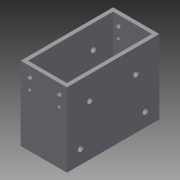
# Autodesk Inventor part: Pitch_Free_Case
Saved by Autodesk Inventor 2013 (Build 170138000, 138)
## iProperties
Created: 2014-05-25
Part Number: Pitch_Free_Case
Material: 一般
Document SubType Name: Modeling
Designer: andou
Density: 1 g/cm^3
Author: andou
Autodesk Inventor part; units mm, degrees
ref_plane "YZ Plane" through (0, 0, 0) normal (1, 0, 0) x (0, 1, 0)
ref_plane "XZ Plane" through (0, 0, 0) normal (0, 1, 0) x (-1, 0, 0)
ref_plane "XY Plane" through (0, 0, 0) normal (0, 0, 1) x (1, 0, 0)
sketch "スケッチ1" plane through (0, 0, 0) normal (0, 0, 1) x (1, 0, 0)
  line L0 (-12.5, 25) -> (12.5, 25)
  line L1 (12.5, 25) -> (12.5, -25)
  line L2 (12.5, -25) -> (-12.5, -25)
  line L3 (-12.5, -25) -> (-12.5, 25)
  line L4 (-10.5, 23) -> (10.5, 23)
  line L5 (10.5, 23) -> (10.5, -23)
  line L6 (10.5, -23) -> (-10.5, -23)
  line L7 (-10.5, -23) -> (-10.5, 23)
  point P0 (0, 0)
  dimension "d0" = 21
  dimension "d2" = 25
  dimension "d3" = 10.5
  dimension "d4" = 46
  dimension "d5" = 50
  dimension "d6" = 23
  dimension "d7" = 25
  dimension "d8" = 12.5
  constraints: 16 end point, 4 parallel, 2 horizontal, 2 perpendicular
  measures "d0" distance of L4.start L4.end
  measures "d2" distance of L0.start L0.end
  measures "d3" distance from line of L7 point (0, 0)
  measures "d4" distance between parallel lines of L6 L4
  measures "d5" distance of L2.end L0.start
  measures "d6" distance from line of point (0, 0) L6
  measures "d7" distance from line of point (0, 0) L2
  measures "d8" distance from line of L1 point (0, 0)
extrude "押し出し1" add sketch "スケッチ1" against normal blind 40
sketch "スケッチ2" plane through (-12.5, 25, 0) normal (0, 1, 0) x (1, 0, 0)
  line L0 (0, 0) -> (25, 0) projected
  line L1 (0, 0) -> (0, 40) projected
  circle A0 centre (4.5, 5) radius 1.5
  circle A1 centre (20.5, 5) radius 1.5
  point P0 (12.5, 0)
  dimension "d13" = 3
  dimension "d14" = 16
  dimension "d16" = 4.5
  dimension "d18" = 5
  dimension "d21" = 5
  constraints: 2 centre point, 1 equal radius
  measures "d13" diameter of A0
  measures "d14" distance of A1.centre A0.centre
  measures "d16" distance from line of L1 A0.centre
  measures "d18" distance from line of L0 A0.centre
  measures "d21" distance from line of A1.centre L0
hole "穴1" at (8, 25, -5) at (-8, 25, -5) direction (0, -1, 0) diameter 3 end through all
sketch "スケッチ3" plane through (-12.5, 25, 0) normal (0, 1, 0) x (1, 0, 0)
  circle A0 centre (20.5, 5) radius 1.5 projected
  circle A1 centre (4.5, 5) radius 1.5 projected
  line L0 (0, 0) -> (0, 40) projected
  circle A2 centre (4.5, 11) radius 1
  circle A3 centre (20.5, 11) radius 1
  point P0 (12.5, 0)
  dimension "d29" = 2
  dimension "d31" = 16
  dimension "d32" = 4.5
  dimension "d33" = 6
  dimension "d34" = 6
  constraints: 2 centre point, 1 equal radius
  measures "d29" diameter of A3
  measures "d31" distance of A3.centre A2.centre
  measures "d32" distance from line of L0 A2.centre
  measures "d33" distance of A2.centre A1.centre
  measures "d34" distance of A3.centre A0.centre
hole "穴2" at (8, 25, -11) at (-8, 25, -11) direction (0, -1, 0) diameter 2 end through all
sketch "スケッチ4" plane through (12.5, -25, 0) normal (1, 0, 0) x (0, 0, -1)
  line L0 (0, 0) -> (40, 0) projected
  line L1 (40, 50) -> (40, 0) projected
  circle A0 centre (32.5, 42.5) radius 1.5
  circle A1 centre (32.5, 7.5) radius 1.5
  circle A2 centre (12.5, 12.5) radius 1.5
  circle A3 centre (12.5, 37.5) radius 1.5
  point P0 (0, 25)
  dimension "d42" = 3
  dimension "d44" = 25
  dimension "d45" = 35
  dimension "d46" = 7.5
  dimension "d47" = 12.5
  dimension "d48" = 20
  dimension "d49" = 20
  dimension "d50" = 7.5
  dimension "d51" = 7.5
  constraints: 4 centre point, 3 equal radius
  measures "d42" diameter of A0
  measures "d44" distance of A3.centre A2.centre
  measures "d45" distance of A0.centre A1.centre
  measures "d46" distance from line of L0 A1.centre
  measures "d47" distance from line of L0 A2.centre
  measures "d48" horizontal distance of A0.centre A3.centre
  measures "d49" horizontal distance of A2.centre A1.centre
  measures "d50" distance from line of L1 A0.centre
  measures "d51" distance from line of L1 A1.centre
hole "穴3" at (12.5, -12.5, -12.5) at (12.5, -17.5, -32.5) at (12.5, 17.5, -32.5) at (12.5, 12.5, -12.5) direction (-1, 0, 0) diameter 3 end through all
